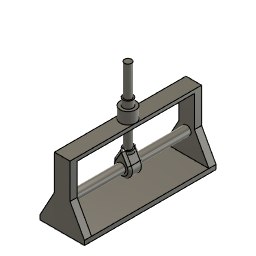
2_Contact (Autodesk Fusion 360 design; units mm, degrees)
Autodesk Fusion 360 part; units mm, degrees
note: some values were not read from the file. Set by a fixed rule: which sketch regions a step uses.
sketch "Sketch1" plane through (0, 0, 0) normal (0, 0, 1) x (1, 0, 0) in component "Shaft"
  circle A0 centre (0, 0) radius 5
  circle A1 centre (0, 0) radius 10
  line L0 (0, 0) -> (0, 15)
  circle A2 centre (0, 15) radius 2.5
  line L1 (-2.1651, 16.25) -> (-8.6603, 5)
  line L2 (2.1651, 16.25) -> (8.6603, 5)
  dimension "d1" = 10
  dimension "d2" = 20
  dimension "d3" = 15
  dimension "d4" = 5
  constraint coincident A0.centre A1.centre
  constraint vertical L0
  constraint coincident L0.end A2.centre
  constraint tangent A2 L1
  constraint tangent A1 L1
  constraint coincident A2 L1.start
  constraint coincident A1 L1.end
  constraint symmetric L0 L1.start L2.start
  constraint symmetric L0 L1.end L2.end
  measures "d1" diameter of A0
  measures "d2" diameter of A1
  measures "d3" distance of A0.centre L0.end
  measures "d4" diameter of A2
sketch "Sketch1 (2)" plane through (0, 0, 0) normal (0, 0, 1) x (1, 0, 0) in component "Frame"
  circle A0 centre (0, 0) radius 10
  line L0 (0, 0) -> (0, -25)
  line L1 (0, -25) -> (-25, -25)
  line L2 (-25, -25) -> (-8.7823, 4.7823)
  line L3 (0, -25) -> (25, -25)
  line L4 (25, -25) -> (8.7823, 4.7823)
  line L5 (-25, -25) -> (25, -25)
  line L6 (25, -25) -> (25, -30)
  line L7 (25, -30) -> (-25, -30)
  line L8 (-25, -30) -> (-25, -25)
  line L9 (-8.7823, 4.7823) -> (-8.7823, 44.0833)
  line L10 (-8.7823, 44.0833) -> (0, 44.0833)
  line L11 (0, 44.0833) -> (0, 10)
  line L12 (8.7823, 4.7823) -> (8.7823, 44.0833)
  line L13 (8.7823, 44.0833) -> (0, 44.0833)
  line L14 (-8.7823, 40.0833) -> (8.7823, 40.0833)
  line L15 (0, 44.0833) -> (0, 40.0833)
  dimension "d9" = 20
  dimension "d22" = 4
  constraint coincident A0.centre L0.start
  constraint vertical L0
  constraint perpendicular L0 L1
  constraint coincident A0 L2.end
  constraint tangent A0 L2
  constraint symmetric L1.start L0 L3.start
  constraint symmetric L0 L1.end L3.end
  constraint symmetric L0 L2.end L4.end
  constraint horizontal L5
  constraint vertical L6
  constraint horizontal L7
  constraint vertical L8
  constraint vertical L9
  constraint perpendicular L9 L10
  constraint coincident A0 L11.end
  constraint perpendicular L10 L11
  constraint symmetric L2.end L11 L4.end
  constraint symmetric L9.end L11 L12.end
  constraint symmetric L10.end L11 L13.end
  constraint coincident L12 L14.end
  constraint perpendicular L12 L14
  constraint coincident L9 L14.start
  constraint midpoint L14 L15.end
  constraint perpendicular L14 L15
  measures "d9" diameter of A0
  measures "d22" distance of L10.end L15.end
extrude "Extrude1" add sketch "Sketch1 (2)" along normal blind 74 and the other way blind -66 makes body 1 in component "Frame"
extrude "Extrude2" add sketch "Sketch1 (2)" along normal blind 74 contours L1 L3 L5 L6 L7 L8 bodies 1 in component "Frame"
mirror "Mirror1" about plane through (0, 0, 0) normal (0, 0, -1) of bodies 1 merged in component "Frame"
extrude "Extrude3" add sketch "Sketch1 (2)" along normal mid plane 132 contours L11 L12 L13 L14 L15 | L9 L10 L11 L14 L15 bodies 1 in component "Frame"
sketch "Sketch2" plane through (0, 44.0833, 0) normal (0, 1, 0) x (-1, 0, 0) in component "Frame"
  line L0 (8.7823, -74) -> (8.7823, 74)
  line L1 (8.7823, 74) -> (-8.7823, 74)
  line L2 (-8.7823, 74) -> (-8.7823, -74)
  line L3 (-8.7823, -74) -> (8.7823, -74)
  circle A0 centre (0, 0) radius 8.7823
  circle A1 centre (0, 0) radius 4
  dimension "d25" = 8
  constraint coincident A0.centre A1.centre
  constraint tangent L0 A0
  constraint concentric A0 A1
  measures "d25" diameter of A1
extrude "Extrude4" add sketch "Sketch2" along normal blind 13 contours A0 bodies 1 in component "Frame"
sketch "Sketch1 (3)" plane through (0, 0, 0) normal (0, 1, 0) x (1, 0, 0) in component "Stab"
  circle A0 centre (0, 0) radius 4
  circle A1 centre (0, 0) radius 5.45
  dimension "d28" = 8
  constraint coincident A0.centre A1.centre
  constraint concentric A0 A1
  measures "d28" diameter of A0
extrude "Extrude1'" add sketch "Sketch1 (3)" along normal blind 100 and the other way blind -14 separate body contours A0 makes body 2 in component "Stab"
extrude "Extrude2'" add sketch "Sketch1 (3)" along normal blind 16 and the other way blind -10 contours A0 | A1 bodies 2 in component "Stab"
fillet "Fillet1" radius 2.5 1 edges at (-5.0812, 10, 1.9708) on bodies 2 in component "Stab"
extrude "Extrude3'" add sketch "Sketch1 (3)" along normal blind 65 and the other way blind -57.083 bodies 2 in component "Stab"
extrude "Extrude3''" add sketch "Sketch1" along normal mid plane 15 separate body makes body 3 in component "Shaft"
extrude "Extrude4'" add sketch "Sketch1" along normal mid plane 132 contours A0 bodies 3 in component "Shaft"
fillet "Fillet1'" radius 2.5 8 edges at (-5.4127, 10.625, 7.5) (0, -10, 7.5) (5.4127, 10.625, 7.5) (0, 17.5, 7.5) (-5.4127, 10.625, -7.5) (0, 17.5, -7.5) (5.4127, 10.625, -7.5) (0, -10, -7.5) on bodies 3 in component "Shaft"
sketch "Sketch4" plane through (0, 0, -66) normal (0, 0, 1) x (1, 0, 0) in component "Frame"
  line L0 (8.7823, 40.0833) -> (-8.7823, 40.0833)
  line L1 (-8.7823, 40.0833) -> (-8.7823, 4.7823)
  line L2 (-8.7823, 4.7823) -> (-25, -25)
  line L3 (-25, -25) -> (25, -25)
  line L4 (25, -25) -> (8.7823, 4.7823)
  line L5 (8.7823, 4.7823) -> (8.7823, 40.0833)
component "Shaft" placed x (1, 0, 0) y (0, 1, 0) z (0, 0, 1) at (0, 0, 0)
component "Frame" placed x (1, 0, 0) y (0, 1, 0) z (0, 0, 1) at (0, 0, 0)
component "Stab" placed x (1, 0, 0) y (0, 1, 0) z (0, 0, 1) at (0, 0, 0)
